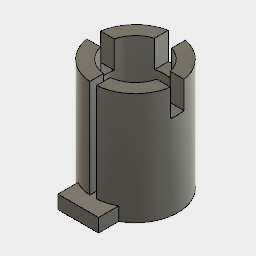
四轴电机支架部件01 (Autodesk Fusion 360 design; units mm, degrees)
Autodesk Fusion 360 part; units mm, degrees
sketch "草图1" plane through (0, 0, 0) normal (0, 1, 0) x (1, 0, 0)
  circle A0 centre (0, 0) radius 4.25
  circle A1 centre (0, 0) radius 1.5
  line L0 (3.0053, -10.45) -> (-2.9947, -10.45)
  line L1 (-2.9947, -10.45) -> (-2.9947, -5.45)
  line L2 (3.0053, -5.45) -> (3.0053, -10.45)
  circle A2 centre (0, 0) radius 6.25
  circle A3 centre (0, 0) radius 3.25
  dimension "d1" = 8.5
  dimension "d3" = 3
  dimension "d5" = 5
  dimension "d6" = 6
  dimension "d7" = 12.5
  dimension "d28" = 6.5
  measures "d1" diameter of A0
  measures "d3" diameter of A1
  measures "d5" distance of L0.end L1.end
  measures "d6" distance of L1.end L2.start
  measures "d7" diameter of A2
  measures "d28" diameter of A3
extrude "拉伸1" add sketch "草图1" along normal blind 17 contours A2
extrude "拉伸2" add sketch "草图1" along normal blind 2 contours L0 L1 L2 A2
extrude "拉伸3" add sketch "草图1" along normal blind 2 contours A0 | A3
sketch "草图3" plane through (0, 17, 0) normal (0, 1, 0) x (-1, 0, 0)
  circle A0 centre (0, 0) radius 4.25
  circle A1 centre (0, 0) radius 6.25
  line L0 (-0.5, 6.75) -> (0.5, 6.75)
  line L1 (0.5, 6.75) -> (0.5, 2.75)
  line L2 (0.5, 2.75) -> (-0.5, 2.75)
  line L3 (-0.5, 2.75) -> (-0.5, 6.75)
  line L4 (-0.5, 6.75) -> (0.5, 2.75) construction
  line L5 (0.5, 6.75) -> (-0.5, 2.75) construction
  point P0 (0, 4.75)
  dimension "d14" = 4
  dimension "d15" = 1
  measures "d14" distance of L0.end L1.end
  measures "d15" distance of L1.end L2.end
extrude "拉伸4" cut sketch "草图3" against normal blind 15 contours A0 A1 L1 L3 picked at (0.389, 4.8991)
sketch "草图4" plane through (0, 2, 0) normal (0, 1, 0) x (-1, 0, 0)
  circle A0 centre (0, 0) radius 1.5
  arc A1 (-0.5, 4.2205) -> (0.5, 4.2205) centre (0, 0) ccw
  line L0 (0.5, 4.2205) -> (0.5, 6.23)
  arc A2 (2.9947, 5.4858) -> (0.5, 6.23) centre (0, 0) ccw
  line L1 (2.9947, 5.4858) -> (2.9947, 10.45)
  line L2 (2.9947, 10.45) -> (-3.0053, 10.45)
  line L3 (-3.0053, 10.45) -> (-3.0053, 5.48)
  arc A3 (-0.5, 6.23) -> (-3.0053, 5.48) centre (0, 0) ccw
  line L4 (-0.5, 6.23) -> (-0.5, 4.2205)
extrude "拉伸6" add 1 faces at (0.8071, 17, 5.5122) along direction (0, 1, 0) blind 5
sketch "草图6" plane through (0, 22, 0) normal (0, 1, 0) x (-1, 0, 0)
  line L0 (-0.5, 4.2205) -> (-0.5, 6.23)
  arc A0 (-0.5, 6.23) -> (0.5, 6.23) centre (0, 0) ccw
  line L1 (0.5, 6.23) -> (0.5, 4.2205)
  arc A1 (-0.5, 4.2205) -> (0.5, 4.2205) centre (0, 0) ccw
  line L2 (-1.2439, -3.8) -> (1.2561, -3.8)
  line L3 (1.2561, -3.8) -> (1.2561, -6.6949)
  line L4 (1.2561, -6.6949) -> (-1.2439, -6.6949)
  line L5 (-1.2439, -6.6949) -> (-1.2439, -3.8)
  line L6 (-1.2439, -3.8) -> (1.2561, -6.6949) construction
  line L7 (1.2561, -3.8) -> (-1.2439, -6.6949) construction
  point P0 (0.0061, -5.2474)
  dimension "d25" = 2.5
  measures "d25" distance of L3.end L4.end
extrude "拉伸7" cut sketch "草图6" against normal blind 3 contours A0 A1 L3 L5
extrude "拉伸8" add sketch "草图1" along normal blind 3.5 contours A0
sketch "草图7" plane through (0, 3.5, 0) normal (0, 1, 0) x (-1, 0, 0)
  circle A0 centre (0, 0) radius 3.25
  arc A1 (-0.5, 4.2205) -> (0.5, 4.2205) centre (0, 0) ccw
  arc A2 (0.5, 4.2205) -> (-0.5, 4.2205) centre (0, 0) ccw
  line L0 (-0.5, 4.6256) -> (0.5, 4.6256)
  line L1 (0.5, 4.6256) -> (0.5, 2.5744)
  line L2 (0.5, 2.5744) -> (-0.5, 2.5744)
  line L3 (-0.5, 2.5744) -> (-0.5, 4.6256)
  line L4 (-0.5, 4.6256) -> (0.5, 2.5744) construction
  line L5 (0.5, 4.6256) -> (-0.5, 2.5744) construction
  line L6 (-0.5, 4.2205) -> (-0.5, 6.23)
  point P0 (0, 3.6)
  dimension "d31" = 1
  measures "d31" distance of L1.end L2.end
extrude "拉伸9" cut sketch "草图7" against normal blind 1.5 contours A0 A2 L1 L3
extrude "拉伸10" add 1 faces at (0.7049, 3.5, 3.8443) along direction (0, 1, 0) blind 1
extrude "拉伸11" cut 2 faces at (-1.5425, 22, -5.3546) (1.5308, 22, -5.358) along direction (0, -1, 0) blind 2.5
extrude "拉伸12" cut 1 faces at (-0.0062, 19, -5.5739) along direction (0, -1, 0) blind 2.5
sketch "草图12" plane through (0, 19.5, 0) normal (0, 1, 0) x (-1, 0, 0)
  line L0 (-1.2439, -6.125) -> (-1.2439, -4.0639)
  arc A0 (-0.5, 4.2205) -> (-1.2439, -4.0639) centre (0, 0) ccw
  line L1 (-0.5, 4.2205) -> (-0.5, 6.23)
  arc A1 (-0.5, 6.23) -> (-1.2439, -6.125) centre (0, 0) ccw
  line L2 (-6.7, 1) -> (-3.7, 1)
  line L3 (-3.7, 1) -> (-3.7, -1)
  line L4 (-3.7, -1) -> (-6.7, -1)
  line L5 (-6.7, -1) -> (-6.7, 1)
  line L6 (-6.7, 1) -> (-3.7, -1) construction
  line L7 (-3.7, 1) -> (-6.7, -1) construction
  line L8 (3.7, 1) -> (6.7, 1)
  line L9 (6.7, 1) -> (6.7, -1)
  line L10 (6.7, -1) -> (3.7, -1)
  line L11 (3.7, -1) -> (3.7, 1)
  line L12 (3.7, 1) -> (6.7, -1) construction
  line L13 (6.7, 1) -> (3.7, -1) construction
  point P0 (-5.2, 0)
  point P1 (5.2, 0)
  dimension "d40" = 2
  dimension "d41" = 2
  measures "d40" distance of L2.end L3.end
  measures "d41" distance of L8.end L9.end
extrude "拉伸13" cut 1 faces at (1.0053, 0.6667, 10.45) along direction (0, 0, -1) blind 2
extrude "拉伸14" cut sketch "草图12" against normal blind 3 contours A0 A1 L2 L4 | L8 L9 L10 L11
extrude "拉伸15" cut 3 faces at (-5.5774, 16.5, 0) (-0.0062, 16.5, -5.5739) (5.5774, 16.5, 0) along direction (0, -1, 0) blind 3
extrude "拉伸16" cut 4 faces at (5.4184, 19.5, 1.2992) (-5.4184, 19.5, 1.2992) (-5.4268, 19.5, -1.2721) (5.4267, 19.5, -1.2726) along direction (0, -1, 0) blind 3
extrude "拉伸17" cut 1 faces at (5.5774, 13.5, 0) along direction (0, -1, 0) blind 1
extrude "拉伸18" cut 1 faces at (-0.0062, 13.5, -5.5739) along direction (0, -1, 0) blind 1
extrude "拉伸19" cut 1 faces at (-5.5774, 13.5, 0) along direction (0, -1, 0) blind 1
extrude "拉伸5" [suppressed]
